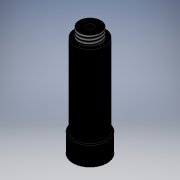
# Autodesk Inventor part: Piston(Deposito_deAceite)
Saved by Autodesk Inventor 2019 (Build 230136000, 136)
## iProperties
Created: 2019-09-21
Part Number: Piston(Deposito_deAceite)
Material: Plástico ABS
Document SubType Name: Modeling
Designer: axelj
Density: 1.06 g/cm^3
Appearance: Anodizado - Negro
Author: axelj
Autodesk Inventor part; units mm, degrees
ref_plane "YZ Plane" through (0, 0, 0) normal (1, 0, 0) x (0, 1, 0)
ref_plane "XZ Plane" through (0, 0, 0) normal (0, 1, 0) x (-1, 0, 0)
ref_plane "XY Plane" through (0, 0, 0) normal (0, 0, 1) x (1, 0, 0)
sketch "Boceto1" plane through (0, 0, 0) normal (0, 1, 0) x (-1, 0, 0)
  circle A0 centre (0, 0) radius 6.05
  dimension "d0" = 12.1
  constraints: 1 centre point, 1 coincident
  measures "d0" diameter of A0
extrude "Extrusión1" add sketch "Boceto1" against normal blind 32.7
sketch "Boceto2" plane through (0, 0, 0) normal (0, 1, 0) x (1, 0, 0)
  circle A0 centre (0, 0) radius 4.35
  dimension "d3" = 8.7
  constraints: 1 centre point, 1 coincident
  measures "d3" diameter of A0
extrude "Extrusión2" add sketch "Boceto2" along normal blind 3.7
thread "Rosca1" size "M9x1.25" class "6g" standard "ANSI Metric M Profile" full length
sketch "Boceto3" plane through (0, -32.7, 0) normal (0, -1, 0) x (1, 0, 0)
  circle A0 centre (0, 0) radius 6.9
  dimension "d8" = 13.8
  constraints: 1 centre point, 1 coincident
  measures "d8" diameter of A0
sketch "Boceto4" plane through (0, -32.7, 0) normal (0, -1, 0) x (1, 0, 0)
  circle A0 centre (0, 0) radius 5.95
  dimension "d9" = 11.9
  constraints: 1 centre point, 1 coincident
  measures "d9" diameter of A0
extrude "Extrusión3" cut sketch "Boceto4" against normal blind 28.7
sketch "Boceto5" plane through (0, -32.7, 0) normal (0, -1, 0) x (1, 0, 0)
  point P0 (0, 0)
extrude "Extrusión4" add sketch "Boceto3" along normal blind 7.6
sketch "Boceto6" plane through (0, 3.7, 0) normal (0, 1, 0) x (1, 0, 0)
  circle A0 centre (0, 0) radius 1.45
  dimension "d14" = 2.9
  constraints: 1 centre point, 1 coincident
  measures "d14" diameter of A0
extrude "Extrusión5" cut sketch "Boceto6" against normal blind 20
sketch "Boceto7" plane through (0, -40.3, 0) normal (0, -1, 0) x (1, 0, 0)
  circle A0 centre (0, 0) radius 6.85
  circle A1 centre (0, 0) radius 6.9
  dimension "d17" = 13.7
  dimension "d18" = 13.8
  constraints: 2 centre point, 2 coincident
  measures "d17" diameter of A0
  measures "d18" diameter of A1
extrude "Extrusión6" cut sketch "Boceto7" against normal blind 20
